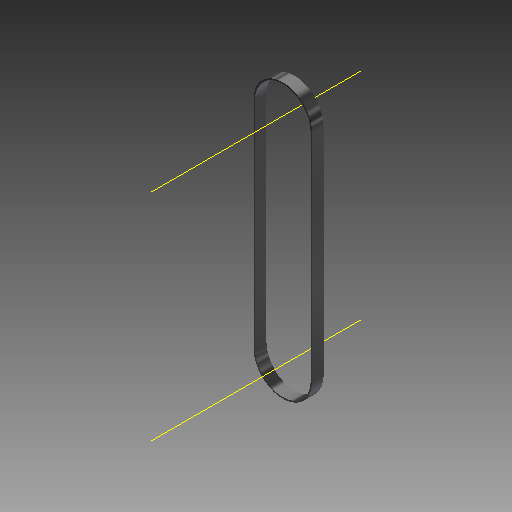
# Autodesk Inventor part: Correia síncrona
Saved by Autodesk Inventor 2018 (Build 220112000, 112)
## iProperties
Created: 2018-09-22
Part Number: Correia síncrona
Material: Rubber
Document SubType Name: Modeling
Designer: Usuario
Density: 1 g/cm^3
Appearance: Rubber - Black - Version 1.1
CustomPartVersion: 1
Author: Usuario
Autodesk Inventor part; units mm, degrees
sketch "Caminho de Esboço" plane through (0, 0, 0) normal (0, 0, 1) x (1, 0, 0)
  arc A0 (-39.7887, 0) -> (39.7887, 0) centre (0, 0) ccw
  arc A1 (39.7887, 300) -> (-39.7887, 300) centre (0, 300) ccw
  line L0 (39.7887, 300) -> (39.7887, 0)
  line L1 (-39.7887, 0) -> (-39.7887, 300)
  constraints: 4 end point, 4 point on circle, 2 centre point
ref_plane "Plano de corte transversal" through (39.7887, 0, 0) normal (0, 1, 0) x (0, 0, 1)
ref_plane "Plano de trabalho2" through (0, 0, 0) normal (-1, 0, 0) x (0, 0, 1)
ref_plane "Plano de trabalho3" through (0, 300, 0) normal (-0.0628, -0.998, 0) x (0, 0, 1)
sketch "Seção transversal" plane through (39.7887, 0, 0) normal (0, 1, 0) x (0, 0, 1)
  line L0 (-8, 1) -> (8, 1)
  line L1 (8, 1) -> (8, -1)
  line L2 (8, -1) -> (-8, -1)
  line L3 (-8, -1) -> (-8, 1)
  line L4 (-8, 0) -> (8, 0) construction
  point P0 (0, 0)
  point P1 (0, 0)
  dimension "d0" = 16
  dimension "d4" = 1
  dimension "d5" = 1
  constraints: 10 end point, 3 midpoint, 2 parallel, 1 coincident, 1 horizontal, 1 perpendicular, 1 other
  measures "d0" distance between parallel lines of L1 L3
  measures "d4" distance between parallel lines of L2 L4
  measures "d5" distance between parallel lines of L4 L0
sweep "Correia" add profiles "Seção transversal" path "Caminho de Esboço"
equation "\"d0\" = da_B"
equation "\"d4\" = da_a"
equation "\"d5\" = da_a2"
equation "\"da_B\" = 16"
equation "\"da_a\" = 1"
equation "\"da_S\" = 5.3"
equation "\"da_Beta\" = 20deg"
equation "\"da_Ht\" = 2.5"
equation "\"da_H\" = 4.5"
equation "\"da_a2\" = 1"
body "Solid1"
